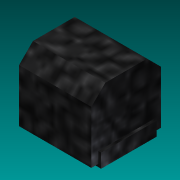
# Autodesk Inventor part: NL565050T-103J-PF
Saved by Autodesk Inventor 2015 (Build 190159000, 159)
## iProperties
Created: 2014-10-18
Part Number: NL565050T-103J-PF
Material: Generic
Document SubType Name: Modeling
Designer: Sawaiz Syed
Density: 1 g/cm^3
Appearance: Black Cast
Author: Sawaiz Syed
Autodesk Inventor part; units mm, degrees
ref_plane "YZ Plane" through (0, 0, 0) normal (1, 0, 0) x (0, 1, 0)
ref_plane "XZ Plane" through (0, 0, 0) normal (0, 1, 0) x (-1, 0, 0)
ref_plane "XY Plane" through (0, 0, 0) normal (0, 0, 1) x (1, 0, 0)
sketch "Sketch1" plane through (0, 0, 0) normal (0, 0, 1) x (1, 0, 0)
  line L0 (-2.8, 2.5) -> (2.8, 2.5)
  line L1 (2.8, 2.5) -> (2.8, -2.5)
  line L2 (2.8, -2.5) -> (-2.8, -2.5)
  line L3 (-2.8, -2.5) -> (-2.8, 2.5)
  line L4 (-2.8, 2.5) -> (2.8, -2.5) construction
  line L5 (2.8, 2.5) -> (-2.8, -2.5) construction
  point P0 (0, 0)
  dimension "d0" = 5.6
  dimension "d1" = 5
  constraints: 12 end point, 2 midpoint, 2 parallel, 1 horizontal, 1 perpendicular
  measures "d0" distance of L1.end L2.end
  measures "d1" distance of L0.end L1.end
extrude "Extrusion1" add sketch "Sketch1" along normal blind 5
chamfer "Chamfer1" distance 1 angle 45 2 edges at (0, -2.5, 5) (0, 2.5, 5)
sketch "Sketch2" plane through (2.8, -2.5, 0) normal (1, 0, 0) x (0, 0, -1)
  line L0 (-5, 4) -> (-4, 5) projected
  line L1 (-5, 1) -> (-5, 4) projected
  line L2 (-4, 0) -> (-5, 1) projected
  line L3 (0, 0) -> (-4, 0) projected
  line L4 (0, 5) -> (0, 0) projected
  line L5 (0, 5) -> (-4, 5) projected
  line L6 (-1, 0.5) -> (0, 0.5)
  line L7 (0, 0.5) -> (0, 4.5)
  line L8 (0, 4.5) -> (-1, 4.5)
  line L9 (-1, 4.5) -> (-1, 0.5)
  point P0 (0, 2.5)
  dimension "d7" = 0.5
  dimension "d8" = 0.5
  dimension "d9" = 1
  constraints: 8 end point, 2 parallel, 1 horizontal, 1 perpendicular, 1 point on line
  measures "d7" distance between parallel lines of L5 L8
  measures "d8" distance between parallel lines of L3 L6
  measures "d9" distance between parallel lines of L4 L9
extrude "Extrusion2" cut sketch "Sketch2" against normal blind 0.2 contours L0 L5 L4 L8 L9 L6 L3 L2 L1
mirror "Mirror1" about plane through (0, 0, 0) normal (1, 0, 0) of "Extrusion2"
sketch "Sketch3" plane through (0, 0, 0) normal (0, 0, -1) x (-1, 0, 0)
  line L0 (2.6, -2.5) -> (2.6, -2) projected
  line L1 (2.6, -2) -> (2.8, -2) projected
  line L2 (2.8, -2) -> (2.8, 2) projected
  line L3 (2.8, 2) -> (2.6, 2) projected
  line L4 (2.6, 2) -> (2.6, 2.5) projected
  line L5 (2.6, 2.5) -> (-2.6, 2.5) projected
  line L6 (-2.6, 2.5) -> (-2.6, 2) projected
  line L7 (-2.6, 2) -> (-2.8, 2) projected
  line L8 (-2.8, 2) -> (-2.8, -2) projected
  line L9 (-2.8, -2) -> (-2.6, -2) projected
  line L10 (-2.6, -2) -> (-2.6, -2.5) projected
  line L11 (-2.6, -2.5) -> (2.6, -2.5) projected
  line L12 (2.8, -2) -> (2.3, -2)
  line L13 (2.3, -2) -> (2.3, 2)
  line L14 (2.3, 2) -> (2.8, 2)
  line L15 (2.8, 2) -> (2.8, -2)
  line L16 (-2.8, -2) -> (-2.3, -2)
  line L17 (-2.3, -2) -> (-2.3, 2)
  line L18 (-2.3, 2) -> (-2.8, 2)
  line L19 (-2.8, 2) -> (-2.8, -2)
  point P0 (0, 0)
  dimension "d12" = 0.5
  dimension "d13" = 4
  dimension "d14" = 0.5
  dimension "d15" = 4
  constraints: 16 end point, 4 parallel, 2 horizontal, 2 perpendicular
  measures "d12" distance of L13.end L14.end
  measures "d13" distance between parallel lines of L1 L14
  measures "d14" distance between parallel lines of L8 L17
  measures "d15" distance between parallel lines of L16 L18
extrude "Extrusion3" cut sketch "Sketch3" against normal blind 0.2 contours L11 L10 L16 L17 L18 L6 L5 L4 L14 L13 L12 L0
equation "\"d14\" = d12"
equation "\"d15\" = d13"
body "Solid1"
